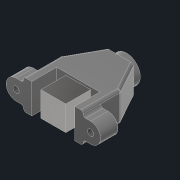
# Autodesk Inventor part: USB2-MBMPAF-XXE
Saved by Autodesk Inventor 2021 (Build 250183000, 183)
## iProperties
Created: 2021-08-05
Part Number: USB2-MBMPAF-XXE
Material: ABS プラスチック
Document SubType Name: Modeling
Designer: yuta0
Density: 1.06 g/cm^3
Appearance: 滑らか - 黒
Author: yuta0
Autodesk Inventor part; units mm, degrees
ref_plane "YZ Plane" through (0, 0, 0) normal (1, 0, 0) x (0, 1, 0)
ref_plane "XZ Plane" through (0, 0, 0) normal (0, 1, 0) x (-1, 0, 0)
ref_plane "XY Plane" through (0, 0, 0) normal (0, 0, 1) x (1, 0, 0)
sketch "スケッチ1" plane through (0, 0, 0) normal (0, 0, 1) x (1, 0, 0)
  line L0 (-12, -6) -> (12, -6)
  line L1 (12, -6) -> (12, 6)
  line L2 (12, 6) -> (-12, 6)
  line L3 (-12, 6) -> (-12, -6)
  line L4 (-12, -6) -> (12, 6) construction
  line L5 (12, -6) -> (-12, 6) construction
  point P0 (0, 0)
  dimension "d0" = 24
  dimension "d1" = 12
  constraints: 12 end point, 2 midpoint, 2 parallel, 1 horizontal, 1 perpendicular
  measures "d0" distance of L1.end L2.end
  measures "d1" distance of L2.end L0.start
extrude "押し出し1" add sketch "スケッチ1" against normal blind 26.7
sketch "スケッチ2" plane through (0, 0, 0) normal (0, 0, 1) x (1, 0, 0)
  line L0 (-15, 0) -> (15, 0) construction
  line L1 (-15, -4) -> (15, -4)
  line L2 (15, 4) -> (-15, 4)
  arc A0 (-15, 4) -> (-15, -4) centre (-15, 0) ccw
  arc A1 (15, -4) -> (15, 4) centre (15, 0) ccw
  point P0 (0, 0)
  dimension "d4" = 30
  dimension "d5" = 4
  constraints: 8 end point, 4 point on circle, 4 tangent, 2 centre point, 1 horizontal, 1 midpoint, 1 parallel
  measures "d4" distance of L0.start L0.end
  measures "d5" radius of A0
extrude "押し出し2" add sketch "スケッチ2" against normal blind 7
sketch "スケッチ3" plane through (0, 0, 0) normal (0, 0, 1) x (1, 0, 0)
  arc A0 (-15, 4) -> (-15, -4) centre (-15, 0) ccw projected
  arc A1 (15, -4) -> (15, 4) centre (15, 0) ccw projected
  point P0 (0, 0)
hole "穴1" at (15, 0, 0) at (-15, 0, 0) direction (0, 0, -1) diameter 2.459 end through all thread size "M3x0.5" class "6H" standard "ANSI Metric M Profile"
sketch "スケッチ4" plane through (0, 0, -26.7) normal (0, 0, -1) x (-1, 0, 0)
  circle A0 centre (0, 0) radius 5.5
  line L0 (12, 6) -> (-12, 6) projected
  dimension "d30" = 11
  constraints: 1 centre point, 1 coincident
  measures "d30" diameter of A0
extrude "押し出し3" add sketch "スケッチ4" along normal blind 2.8
sketch "スケッチ5" plane through (-12, 6, 0) normal (0, 1, 0) x (1, 0, 0)
  line L0 (17.5, 29.5) -> (6.5, 29.5) projected
  line L1 (6.5, 26.7) -> (17.5, 26.7) projected
  line L2 (6.5, 26.7) -> (17.5, 26.7) projected
  line L3 (6.5, 26.7) -> (6.5, 26.7) projected
  line L4 (17.5, 26.7) -> (24, 15)
  line L5 (24, 0) -> (24, 26.7) projected
  line L6 (24, 0) -> (0, 0) projected
  line L7 (6.5, 26.7) -> (0, 15)
  line L8 (0, 0) -> (0, 26.7) projected
  line L9 (24, 0) -> (0, 0) projected
  line L10 (24, 0) -> (24, 26.7) projected
  line L11 (0, 26.7) -> (24, 26.7) projected
  line L12 (0, 0) -> (0, 26.7) projected
  point P0 (12, 0)
  point P1 (17.5, 26.7)
  point P2 (6.5, 26.7)
  dimension "d18" = 15
  dimension "d19" = 15
  constraints: 4 end point, 2 point on line
  measures "d18" distance from line of L6 L4.end
  measures "d19" distance from line of L6 L7.end
extrude "押し出し4" cut sketch "スケッチ5" against normal through all contours L7 L8 L11 | L11 L5 L4
sketch "スケッチ6" plane through (0, 0, 0) normal (0, 0, 1) x (1, 0, 0)
  line L0 (-8.65, -6) -> (8.65, -6)
  line L1 (8.65, -6) -> (8.65, 6)
  line L2 (8.65, 6) -> (-8.65, 6)
  line L3 (-8.65, 6) -> (-8.65, -6)
  line L4 (-8.65, -6) -> (8.65, 6) construction
  line L5 (8.65, -6) -> (-8.65, 6) construction
  line L6 (12, 6) -> (-12, 6) projected
  point P0 (0, 0)
  dimension "d22" = 17.3
  constraints: 12 end point, 2 midpoint, 2 parallel, 1 horizontal, 1 perpendicular, 1 point on line
  measures "d22" distance between parallel lines of L3 L1
extrude "押し出し5" cut sketch "スケッチ6" against normal blind 10
sketch "スケッチ7" plane through (0, 0, -10) normal (0, 0, 1) x (1, 0, 0)
  line L0 (-5, -5) -> (5, -5)
  line L1 (5, -5) -> (5, 5)
  line L2 (5, 5) -> (-5, 5)
  line L3 (-5, 5) -> (-5, -5)
  line L4 (-5, -5) -> (5, 5) construction
  line L5 (5, -5) -> (-5, 5) construction
  point P0 (0, 0)
  dimension "d25" = 10
  dimension "d26" = 10
  constraints: 12 end point, 2 midpoint, 2 parallel, 1 horizontal, 1 perpendicular
  measures "d25" distance of L2.end L1.end
  measures "d26" distance of L1.end L0.end
extrude "押し出し6" add sketch "スケッチ7" along normal blind 10
fillet "フィレット1" radius 1 14 edges at (12, 4, -3.5) (12, -4, -3.5) (-12, -4, -3.5) (-12, -6, -7.5) (12, -6, -7.5) (12, 6, -7.5) (-12, 4, -3.5) (-12, 6, -7.5) (-8.75, 6, -20.85) (-12, 0, -15) (-8.75, -6, -20.85) (8.75, -6, -20.85) (12, 0, -15) (8.75, 6, -20.85)
